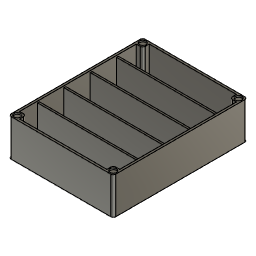
Wingspan - Food Tokens Container (Autodesk Fusion 360 design; units mm, degrees)
Autodesk Fusion 360 part; units mm, degrees
sketch "Skizze1" plane through (0, 0, 0) normal (0, 0, 1) x (1, 0, 0)
  line L0 (0, 0) -> (85, 0)
  line L1 (85, 0) -> (85, 109)
  line L2 (85, 109) -> (0, 109)
  line L3 (0, 109) -> (0, 0)
  dimension "d1" = 85
  dimension "d2" = 109
  constraint horizontal L0
  constraint vertical L1
  constraint horizontal L2
  constraint vertical L3
  constraint coincident L0.start L3.end
  measures "d1" distance of L0.start L0.end
  measures "d2" distance of L0.start L2.end
extrude "Extrusion11" add sketch "Skizze1" along normal blind 30
sketch "Skizze7" plane through (0, 0, 30) normal (0, 0, 1) x (-1, 0, 0)
  line L0 (0, -109) -> (0, 0)
  line L1 (0, 0) -> (-85, 0)
  line L2 (-85, 0) -> (-85, -109)
  line L3 (-85, -109) -> (0, -109)
  line L4 (0, -109) -> (-7, -109)
  line L5 (-7, -109) -> (-7, -102)
  line L6 (-7, -102) -> (0, -102)
  line L7 (0, -102) -> (0, -109)
  line L8 (-85, -109) -> (-78, -109)
  line L9 (-78, -109) -> (-78, -102)
  line L10 (-78, -102) -> (-85, -102)
  line L11 (-85, -102) -> (-85, -109)
  line L12 (0, 0) -> (-7, 0)
  line L13 (-7, 0) -> (-7, -7)
  line L14 (-7, -7) -> (0, -7)
  line L15 (0, -7) -> (0, 0)
  line L16 (-85, 0) -> (-78, 0)
  line L17 (-78, 0) -> (-78, -7)
  line L18 (-78, -7) -> (-85, -7)
  line L19 (-85, -7) -> (-85, 0)
  circle A0 centre (-3.5, -3.5) radius 2.65
  circle A1 centre (-81.5, -3.5) radius 2.65
  circle A2 centre (-81.5, -105.5) radius 2.65
  circle A3 centre (-3.5, -105.5) radius 2.65
  dimension "d103" = 7
  dimension "d104" = 7
  dimension "d105" = 7
  dimension "d106" = 7
  dimension "d107" = 7
  dimension "d108" = 7
  dimension "d109" = 7
  dimension "d110" = 7
  dimension "d111" = 5.3
  dimension "d112" = 5.3
  dimension "d113" = 5.3
  dimension "d114" = 5.3
  dimension "d115" = 3.5
  dimension "d116" = 3.5
  dimension "d117" = 3.5
  dimension "d118" = 3.5
  dimension "d119" = 3.5
  dimension "d120" = 3.5
  dimension "d121" = 3.5
  dimension "d122" = 3.5
  constraint horizontal L4
  constraint vertical L5
  constraint horizontal L6
  constraint vertical L7
  constraint coincident L0.start L3.end
  constraint horizontal L8
  constraint vertical L9
  constraint horizontal L10
  constraint vertical L11
  constraint coincident L2.end L3.start
  constraint horizontal L12
  constraint vertical L13
  constraint horizontal L14
  constraint vertical L15
  constraint coincident L0.end L1.start
  constraint horizontal L16
  constraint vertical L17
  constraint horizontal L18
  constraint vertical L19
  constraint coincident L1.end L2.start
  measures "d103" distance of L0.start L4.end
  measures "d104" distance of L0.start L6.end
  measures "d105" distance of L2.end L8.end
  measures "d106" distance of L2.end L10.end
  measures "d107" distance of L0.end L12.end
  measures "d108" distance of L0.end L14.end
  measures "d109" distance of L1.end L16.end
  measures "d110" distance of L1.end L18.end
  measures "d111" diameter of A0
  measures "d112" diameter of A1
  measures "d113" diameter of A2
  measures "d114" diameter of A3
  measures "d115" distance of L7 A3.centre
  measures "d116" distance of L4 A3.centre
  measures "d117" distance of L11 A2.centre
  measures "d118" distance of L8 A2.centre
  measures "d119" distance of L19 A1.centre
  measures "d120" distance of L18 A1.centre
  measures "d121" distance of L14 A0.centre
  measures "d122" distance of L15 A0.centre
extrude "Extrusion12" cut sketch "Skizze7" against normal blind 1.2 contours A0 | A1 | A2 | A3
sketch "Skizze8" plane through (0, 0, 30) normal (0, 0, 1) x (-1, 0, 0)
  circle A0 centre (-81.5, -3.5) radius 2.65
  circle A1 centre (-3.5, -105.5) radius 2.65
  circle A2 centre (-3.5, -3.5) radius 2.65
  circle A3 centre (-81.5, -105.5) radius 2.65
  line L0 (0, -109) -> (0, 0)
  line L1 (0, 0) -> (-85, 0)
  line L2 (-85, 0) -> (-85, -109)
  line L3 (-85, -109) -> (0, -109)
  line L4 (-7, -1.75) -> (-78, -1.75)
  line L5 (-78, -1.75) -> (-78, -107.25)
  line L6 (-78, -107.25) -> (-7, -107.25)
  line L7 (-7, -107.25) -> (-7, -1.75)
  line L8 (-85, -109) -> (0, -109)
  line L9 (-7, -102) -> (-1.75, -102)
  line L10 (-1.75, -102) -> (-1.75, -7)
  line L11 (-1.75, -7) -> (-7, -7)
  line L12 (-7, -7) -> (-7, -102)
  line L13 (0, 0) -> (-7, 0)
  line L14 (0, -109) -> (-7, -109)
  line L15 (-78, -7) -> (-83.25, -7)
  line L16 (-83.25, -7) -> (-83.25, -102)
  line L17 (-83.25, -102) -> (-78, -102)
  line L18 (-78, -102) -> (-78, -7)
  line L19 (-85, 0) -> (-85, -109)
  line L20 (-85, -109) -> (-78, -109)
  line L21 (-85, 0) -> (-78, 0)
  dimension "d125" = 1.75
  dimension "d126" = 7
  dimension "d127" = 7
  dimension "d128" = 1.75
  dimension "d129" = 1.75
  dimension "d130" = 7
  dimension "d131" = 7
  dimension "d132" = 1.75
  dimension "d133" = 7
  dimension "d134" = 7
  constraint horizontal L4
  constraint vertical L5
  constraint horizontal L6
  constraint vertical L7
  constraint horizontal L9
  constraint vertical L10
  constraint horizontal L11
  constraint vertical L12
  constraint coincident L7 L9.start
  constraint horizontal L15
  constraint vertical L16
  constraint horizontal L17
  constraint vertical L18
  constraint coincident L5 L15.start
  measures "d125" distance of L1 L4
  measures "d126" distance of L0 L7
  measures "d127" distance of L2 L5
  measures "d128" distance of L6 L8
  measures "d129" distance of L0 L10
  measures "d130" distance of L11 L13
  measures "d131" distance of L9 L14
  measures "d132" distance of L16 L19
  measures "d133" distance of L17 L20
  measures "d134" distance of L15 L21
extrude "Extrusion13" cut sketch "Skizze8" against normal blind 28.25 contours L4 L5 L6 L7 L12 L18 | L7 L9 L10 L11 L12 | L5 L15 L16 L17 L18
sketch "Skizze9" plane through (0, 0, 0) normal (0, 0, -1) x (1, 0, 0)
  line L0 (0, 0) -> (0, -109)
  line L1 (0, -109) -> (85, -109)
  line L2 (85, -109) -> (85, 0)
  line L3 (85, 0) -> (0, 0)
  line L4 (0, 0) -> (7, 0)
  line L5 (7, 0) -> (7, -7)
  line L6 (7, -7) -> (0, -7)
  line L7 (0, -7) -> (0, 0)
  line L8 (85, 0) -> (78, 0)
  line L9 (78, 0) -> (78, -7)
  line L10 (78, -7) -> (85, -7)
  line L11 (85, -7) -> (85, 0)
  line L12 (85, -109) -> (78, -109)
  line L13 (78, -109) -> (78, -102)
  line L14 (78, -102) -> (85, -102)
  line L15 (85, -102) -> (85, -109)
  line L16 (0, -109) -> (7, -109)
  line L17 (7, -109) -> (7, -102)
  line L18 (7, -102) -> (0, -102)
  line L19 (0, -102) -> (0, -109)
  circle A0 centre (3.5, -105.5) radius 2.65
  circle A1 centre (81.5, -105.5) radius 2.65
  circle A2 centre (81.5, -3.5) radius 2.65
  circle A3 centre (3.5, -3.5) radius 2.65
  dimension "d137" = 7
  dimension "d138" = 7
  dimension "d139" = 7
  dimension "d140" = 7
  dimension "d141" = 7
  dimension "d142" = 7
  dimension "d143" = 7
  dimension "d144" = 7
  dimension "d145" = 5.3
  dimension "d146" = 3.5
  dimension "d147" = 3.5
  dimension "d148" = 5.3
  dimension "d149" = 3.5
  dimension "d150" = 3.5
  dimension "d151" = 5.3
  dimension "d152" = 3.5
  dimension "d153" = 3.5
  dimension "d154" = 5.3
  dimension "d155" = 3.5
  dimension "d156" = 3.5
  constraint horizontal L4
  constraint vertical L5
  constraint horizontal L6
  constraint vertical L7
  constraint coincident L0.start L3.end
  constraint horizontal L8
  constraint vertical L9
  constraint horizontal L10
  constraint vertical L11
  constraint coincident L2.end L3.start
  constraint horizontal L12
  constraint vertical L13
  constraint horizontal L14
  constraint vertical L15
  constraint coincident L1.end L2.start
  constraint horizontal L16
  constraint vertical L17
  constraint horizontal L18
  constraint vertical L19
  constraint coincident L0.end L1.start
  measures "d137" distance of L0.start L4.end
  measures "d138" distance of L0.start L6.end
  measures "d139" distance of L2.end L8.end
  measures "d140" distance of L2.end L10.end
  measures "d141" distance of L1.end L12.end
  measures "d142" distance of L1.end L14.end
  measures "d143" distance of L0.end L16.end
  measures "d144" distance of L0.end L18.end
  measures "d145" diameter of A0
  measures "d146" distance of L16 A0.centre
  measures "d147" distance of L19 A0.centre
  measures "d148" diameter of A1
  measures "d149" distance of L12 A1.centre
  measures "d150" distance of L15 A1.centre
  measures "d151" diameter of A2
  measures "d152" distance of L11 A2.centre
  measures "d153" distance of L8 A2.centre
  measures "d154" diameter of A3
  measures "d155" distance of L4 A3.centre
  measures "d156" distance of L7 A3.centre
extrude "Extrusion14" cut sketch "Skizze9" against normal blind 1.2 contours A0 | A1 | A2 | A3
sketch "Skizze10" plane through (0, 0, 1.75) normal (0, 0, 1) x (-1, 0, 0)
  line L0 (-83.25, -102) -> (-78, -102)
  line L1 (-78, -102) -> (-78, -107.25)
  line L2 (-78, -107.25) -> (-7, -107.25)
  line L3 (-7, -107.25) -> (-7, -102)
  line L4 (-7, -102) -> (-1.75, -102)
  line L5 (-1.75, -102) -> (-1.75, -7)
  line L6 (-1.75, -7) -> (-7, -7)
  line L7 (-7, -7) -> (-7, -1.75)
  line L8 (-7, -1.75) -> (-78, -1.75)
  line L9 (-78, -1.75) -> (-78, -7)
  line L10 (-78, -7) -> (-83.25, -7)
  line L11 (-83.25, -7) -> (-83.25, -102)
  line L12 (-83.25, -87.35) -> (-1.75, -87.35)
  line L13 (-1.75, -87.35) -> (-1.75, -85.85)
  line L14 (-1.75, -85.85) -> (-83.25, -85.85)
  line L15 (-83.25, -85.85) -> (-83.25, -87.35)
  line L16 (-83.25, -65.95) -> (-1.75, -65.95)
  line L17 (-1.75, -65.95) -> (-1.75, -64.45)
  line L18 (-1.75, -64.45) -> (-83.25, -64.45)
  line L19 (-83.25, -64.45) -> (-83.25, -65.95)
  line L20 (-83.25, -44.55) -> (-1.75, -44.55)
  line L21 (-1.75, -44.55) -> (-1.75, -43.05)
  line L22 (-1.75, -43.05) -> (-83.25, -43.05)
  line L23 (-83.25, -43.05) -> (-83.25, -44.55)
  line L24 (-83.25, -23.15) -> (-1.75, -23.15)
  line L25 (-1.75, -23.15) -> (-1.75, -21.65)
  line L26 (-1.75, -21.65) -> (-83.25, -21.65)
  line L27 (-83.25, -21.65) -> (-83.25, -23.15)
  dimension "d159" = 1.5
  dimension "d160" = 19.9
  dimension "d161" = 1.5
  dimension "d162" = 19.9
  dimension "d163" = 1.5
  dimension "d164" = 19.9
  dimension "d165" = 1.5
  dimension "d166" = 19.9
  constraint horizontal L12
  constraint vertical L13
  constraint horizontal L14
  constraint vertical L15
  constraint coincident L5 L13.end
  constraint coincident L11 L12.start
  constraint horizontal L16
  constraint vertical L17
  constraint horizontal L18
  constraint vertical L19
  constraint coincident L5 L17.end
  constraint coincident L11 L16.start
  constraint horizontal L20
  constraint vertical L21
  constraint horizontal L22
  constraint vertical L23
  constraint coincident L5 L21.end
  constraint coincident L11 L20.start
  constraint horizontal L24
  constraint vertical L25
  constraint horizontal L26
  constraint vertical L27
  constraint coincident L5 L25.end
  constraint coincident L11 L24.start
  measures "d159" distance of L12 L14
  measures "d160" distance of L2 L12
  measures "d161" distance of L16 L18
  measures "d162" distance of L14 L16
  measures "d163" distance of L20 L22
  measures "d164" distance of L18 L20
  measures "d165" distance of L24 L26
  measures "d166" distance of L22 L24
extrude "Extrusion15" add sketch "Skizze10" along normal blind 27 contours L5 L11 L12 L13 L14 L15 | L5 L11 L16 L17 L18 L19 | L5 L11 L20 L21 L22 L23 | L5 L11 L24 L25 L26 L27
fillet "Abrundung4" radius 2 8 edges at (0, 109, 15) (0, 0, 15) (85, 0, 15) (85, 109, 15) (7, 102, 15.875) (7, 7, 15.875) (78, 7, 15.875) (78, 102, 15.875)
sketch "Skizze11" plane through (0, 0, 1.75) normal (0, 0, 1) x (-1, 0, 0)
  line L0 (-83.25, -21.65) -> (-1.75, -21.65)
  line L1 (-1.75, -21.65) -> (-1.75, -7)
  line L2 (-1.75, -7) -> (-5, -7)
  arc A0 (-7, -5) -> (-5, -7) centre (-5, -5) ccw
  line L3 (-7, -5) -> (-7, -1.75)
  line L4 (-7, -1.75) -> (-78, -1.75)
  line L5 (-78, -1.75) -> (-78, -5)
  arc A1 (-80, -7) -> (-78, -5) centre (-80, -5) ccw
  line L6 (-80, -7) -> (-83.25, -7)
  line L7 (-83.25, -7) -> (-83.25, -21.65)
  spline S0 degree 3 poles (-39.178, -19.5242) (-39.2616, -19.4406) (-39.167, -18.9822) (-38.9679, -18.5054) knots 0 0 0 0 1 1 1 1
  line L8 (-38.9679, -18.5054) -> (-38.6057, -17.6386)
  line L9 (-38.6057, -17.6386) -> (-39.8375, -16.3539)
  spline S1 degree 3 poles (-39.8375, -16.3539) (-41.1646, -14.9699) (-42.027, -14.6539) (-44.5452, -14.6292) knots 0 0 0 0 1 1 1 1
  spline S2 degree 3 poles (-44.5452, -14.6292) (-48.426, -14.5911) (-50.326, -12.4607) (-50.3212, -8.1525) knots 0 0 0 0 1 1 1 1
  spline S3 degree 3 poles (-50.3212, -8.1525) (-50.3184, -5.5992) (-49.8967, -4.7798) (-48.5851, -4.7798) knots 0 0 0 0 1 1 1 1
  spline S4 degree 3 poles (-48.5851, -4.7798) (-47.4873, -4.7798) (-47.295, -5.142) (-47.1328, -7.5151) knots 0 0 0 0 1 1 1 1
  spline S5 degree 3 poles (-47.1328, -7.5151) (-47.0433, -8.8234) (-46.8587, -9.5644) (-46.5038, -10.0381) knots 0 0 0 0 1 1 1 1
  spline S6 degree 3 poles (-46.5038, -10.0381) (-46.014, -10.6921) (-45.9327, -10.709) (-43.2549, -10.7115) knots 0 0 0 0 1 1 1 1
  spline S7 degree 3 poles (-43.2549, -10.7115) (-40.9745, -10.7136) (-40.3063, -10.8069) (-39.3182, -11.2613) knots 0 0 0 0 1 1 1 1
  spline S8 degree 3 poles (-39.3182, -11.2613) (-38.0099, -11.8629) (-35.6932, -13.8922) (-35.4539, -14.6461) knots 0 0 0 0 1 1 1 1
  spline S9 degree 3 poles (-35.4539, -14.6461) (-35.335, -15.0207) (-35.0599, -15.1242) (-34.1837, -15.1242) knots 0 0 0 0 1 1 1 1
  spline S10 degree 3 poles (-34.1837, -15.1242) (-33.3782, -15.1242) (-33.0654, -15.2259) (-33.0654, -15.4878) knots 0 0 0 0 1 1 1 1
  spline S11 degree 3 poles (-33.0654, -15.4878) (-33.0654, -15.9956) (-33.5581, -16.2462) (-33.8947, -15.9096) knots 0 0 0 0 1 1 1 1
  spline S12 degree 3 poles (-33.8947, -15.9096) (-34.2764, -15.5279) (-35.3348, -15.5533) (-35.3417, -15.9442) knots 0 0 0 0 1 1 1 1
  spline S13 degree 3 poles (-35.3417, -15.9442) (-35.3541, -16.6404) (-36.2962, -17.4664) (-37.255, -17.6217) knots 0 0 0 0 1 1 1 1
  spline S14 degree 3 poles (-37.255, -17.6217) (-38.1386, -17.7648) (-38.2503, -17.8673) (-38.3638, -18.6401) knots 0 0 0 0 1 1 1 1
  spline S15 degree 3 poles (-38.3638, -18.6401) (-38.4838, -19.4576) (-38.8486, -19.8537) (-39.178, -19.5242) knots 0 0 0 0 1 1 1 1
  spline S16 degree 3 poles (-48.0381, -37.5695) (-47.8963, -37.326) (-47.5089, -37.1504) (-47.1139, -37.1504) knots 0 0 0 0 1 1 1 1
  spline S17 degree 3 poles (-47.1139, -37.1504) (-46.1113, -37.1504) (-45.5008, -37.8028) (-44.8901, -39.527) knots 0 0 0 0 1 1 1 1
  spline S18 degree 3 poles (-44.8901, -39.527) (-44.5903, -40.3731) (-44.2177, -41.1071) (-44.062, -41.1581) knots 0 0 0 0 1 1 1 1
  spline S19 degree 3 poles (-44.062, -41.1581) (-43.5866, -41.3138) (-43.2627, -40.3632) (-43.4171, -39.2653) knots 0 0 0 0 1 1 1 1
  spline S20 degree 3 poles (-43.4171, -39.2653) (-43.5316, -38.4508) (-43.7224, -38.1252) (-44.3057, -37.7491) knots 0 0 0 0 1 1 1 1
  spline S21 degree 3 poles (-44.3057, -37.7491) (-45.5367, -36.9552) (-46.1328, -35.6221) (-46.1374, -33.653) knots 0 0 0 0 1 1 1 1
  spline S22 degree 3 poles (-46.1374, -33.653) (-46.1395, -32.7173) (-46.0712, -31.281) (-45.9855, -30.4612) knots 0 0 0 0 1 1 1 1
  spline S23 degree 3 poles (-45.9855, -30.4612) (-45.8497, -29.1622) (-45.7724, -28.9856) (-45.3837, -29.0873) knots 0 0 0 0 1 1 1 1
  spline S24 degree 3 poles (-45.3837, -29.0873) (-44.801, -29.2397) (-44.6054, -28.8388) (-44.089, -26.4331) knots 0 0 0 0 1 1 1 1
  spline S25 degree 3 poles (-44.089, -26.4331) (-43.7861, -25.0222) (-43.5619, -24.4573) (-43.3046, -24.4573) knots 0 0 0 0 1 1 1 1
  spline S26 degree 3 poles (-43.3046, -24.4573) (-43.1065, -24.4573) (-42.128, -25.2386) (-41.1301, -26.1936) knots 0 0 0 0 1 1 1 1
  spline S27 degree 3 poles (-41.1301, -26.1936) (-39.2398, -28.0026) (-38.815, -28.9068) (-39.874, -28.8668) knots 0 0 0 0 1 1 1 1
  spline S28 degree 3 poles (-39.874, -28.8668) (-40.3813, -28.8476) (-40.4184, -28.9198) (-40.2801, -29.6571) knots 0 0 0 0 1 1 1 1
  spline S29 degree 3 poles (-40.2801, -29.6571) (-40.1963, -30.1034) (-39.8643, -30.9641) (-39.5422, -31.5699) knots 0 0 0 0 1 1 1 1
  spline S30 degree 3 poles (-39.5422, -31.5699) (-38.8325, -32.9048) (-38.7828, -34.4696) (-39.4067, -35.8431) knots 0 0 0 0 1 1 1 1
  spline S31 degree 3 poles (-39.4067, -35.8431) (-39.916, -36.9641) (-41.1366, -38.0773) (-42.0588, -38.2618) knots 0 0 0 0 1 1 1 1
  spline S32 degree 3 poles (-42.0588, -38.2618) (-42.6091, -38.3718) (-42.6849, -38.4878) (-42.5972, -39.0857) knots 0 0 0 0 1 1 1 1
  spline S33 degree 3 poles (-42.5972, -39.0857) (-42.4138, -40.3352) (-42.7591, -41.4619) (-43.4, -41.7056) knots 0 0 0 0 1 1 1 1
  spline S34 degree 3 poles (-43.4, -41.7056) (-44.4841, -42.1177) (-45.0821, -41.6481) (-45.6512, -39.9379) knots 0 0 0 0 1 1 1 1
  spline S35 degree 3 poles (-45.6512, -39.9379) (-46.2604, -38.1073) (-46.6824, -37.6428) (-47.355, -38.0629) knots 0 0 0 0 1 1 1 1
  spline S36 degree 3 poles (-47.355, -38.0629) (-48.2118, -38.598) (-48.5112, -38.3817) (-48.0381, -37.5695) knots 0 0 0 0 1 1 1 1
sketch "Skizze12" plane through (0, 0, 1.75) normal (0, 0, 1) x (-1, 0, 0)
  line L0 (-1.75, -44.55) -> (-83.25, -44.55)
  line L1 (-83.25, -44.55) -> (-83.25, -64.45)
  line L2 (-83.25, -64.45) -> (-1.75, -64.45)
  line L3 (-1.75, -64.45) -> (-1.75, -44.55)
  spline S0 degree 3 poles (-49.7706, -52.9271) (-49.2736, -51.3545) (-48.2065, -50.5145) (-46.7263, -50.5306) knots 0 0 0 0 1 1 1 1
  spline S1 degree 3 poles (-46.7263, -50.5306) (-45.7005, -50.5418) (-44.2379, -51.4293) (-43.9023, -52.2442) knots 0 0 0 0 1 1 1 1
  spline S2 degree 3 poles (-43.9023, -52.2442) (-43.6832, -52.7759) (-43.4579, -52.8987) (-42.4991, -53.0086) knots 0 0 0 0 1 1 1 1
  spline S3 degree 3 poles (-42.4991, -53.0086) (-41.8709, -53.0806) (-41.1277, -53.2147) (-40.8474, -53.3066) knots 0 0 0 0 1 1 1 1
  spline S4 degree 3 poles (-40.8474, -53.3066) (-40.4432, -53.4391) (-40.3494, -53.4082) (-40.3937, -53.157) knots 0 0 0 0 1 1 1 1
  spline S5 degree 3 poles (-40.3937, -53.157) (-40.4245, -52.9828) (-40.7763, -52.7679) (-41.1755, -52.6793) knots 0 0 0 0 1 1 1 1
  spline S6 degree 3 poles (-41.1755, -52.6793) (-42.9496, -52.286) (-43.954, -50.4074) (-43.2546, -48.7907) knots 0 0 0 0 1 1 1 1
  spline S7 degree 3 poles (-43.2546, -48.7907) (-42.4335, -46.8925) (-40.0051, -46.522) (-38.6625, -48.0901) knots 0 0 0 0 1 1 1 1
  spline S8 degree 3 poles (-38.6625, -48.0901) (-37.654, -49.268) (-37.9063, -51.2765) (-39.1693, -52.1244) knots 0 0 0 0 1 1 1 1
  spline S9 degree 3 poles (-39.1693, -52.1244) (-40.1579, -52.7881) (-39.8896, -53.4953) (-38.2085, -54.6568) knots 0 0 0 0 1 1 1 1
  spline S10 degree 3 poles (-38.2085, -54.6568) (-36.6829, -55.7109) (-34.4155, -58.5444) (-34.5488, -59.2304) knots 0 0 0 0 1 1 1 1
  spline S11 degree 3 poles (-34.5488, -59.2304) (-34.7584, -60.3092) (-35.9602, -59.9491) (-36.1778, -58.7423) knots 0 0 0 0 1 1 1 1
  spline S12 degree 3 poles (-36.1778, -58.7423) (-36.2345, -58.4273) (-36.6207, -57.6838) (-37.0358, -57.0901) knots 0 0 0 0 1 1 1 1
  spline S13 degree 3 poles (-37.0358, -57.0901) (-37.6472, -56.216) (-37.8956, -56.0292) (-38.3427, -56.108) knots 0 0 0 0 1 1 1 1
  spline S14 degree 3 poles (-38.3427, -56.108) (-39.3574, -56.287) (-39.5439, -56.5254) (-39.2742, -57.2992) knots 0 0 0 0 1 1 1 1
  spline S15 degree 3 poles (-39.2742, -57.2992) (-38.7276, -58.8673) (-39.8079, -60.5236) (-41.5812, -60.8363) knots 0 0 0 0 1 1 1 1
  spline S16 degree 3 poles (-41.5812, -60.8363) (-42.3513, -60.9721) (-42.6827, -60.8888) (-43.4169, -60.3747) knots 0 0 0 0 1 1 1 1
  spline S17 degree 3 poles (-43.4169, -60.3747) (-44.206, -59.8222) (-44.3372, -59.6086) (-44.5181, -58.5827) knots 0 0 0 0 1 1 1 1
  spline S18 degree 3 poles (-44.5181, -58.5827) (-44.699, -57.5567) (-44.6487, -57.3112) (-44.0962, -56.522) knots 0 0 0 0 1 1 1 1
  spline S19 degree 3 poles (-44.0962, -56.522) (-43.561, -55.7578) (-43.3145, -55.599) (-42.4179, -55.4409) knots 0 0 0 0 1 1 1 1
  spline S20 degree 3 poles (-42.4179, -55.4409) (-41.7308, -55.3197) (-41.1571, -55.3679) (-40.7612, -55.5801) knots 0 0 0 0 1 1 1 1
  spline S21 degree 3 poles (-40.7612, -55.5801) (-40.1874, -55.8876) (-39.1508, -55.7318) (-38.9839, -55.3129) knots 0 0 0 0 1 1 1 1
  spline S22 degree 3 poles (-38.9839, -55.3129) (-38.8763, -55.0427) (-40.8372, -54.2918) (-42.1581, -54.0974) knots 0 0 0 0 1 1 1 1
  spline S23 degree 3 poles (-42.1581, -54.0974) (-43.079, -53.9618) (-43.3643, -53.9892) (-43.398, -54.2163) knots 0 0 0 0 1 1 1 1
  spline S24 degree 3 poles (-43.398, -54.2163) (-43.4976, -54.8884) (-44.5427, -56.2674) (-45.2338, -56.639) knots 0 0 0 0 1 1 1 1
  spline S25 degree 3 poles (-45.2338, -56.639) (-47.6852, -57.957) (-50.6052, -55.5679) (-49.7706, -52.9271) knots 0 0 0 0 1 1 1 1
  spline S26 degree 3 poles (-45.2787, -74.9924) (-44.9999, -74.3782) (-44.3971, -73.3538) (-43.9391, -72.716) knots 0 0 0 0 1 1 1 1
  line L4 (-43.9391, -72.716) -> (-43.1064, -71.5565)
  line L5 (-43.1064, -71.5565) -> (-43.5424, -70.1731)
  spline S27 degree 3 poles (-43.5424, -70.1731) (-44.2718, -67.8593) (-44.0313, -66.6033) (-43.0637, -67.6725) knots 0 0 0 0 1 1 1 1
  spline S28 degree 3 poles (-43.0637, -67.6725) (-42.5023, -68.2929) (-42.1203, -68.313) (-41.0839, -67.7771) knots 0 0 0 0 1 1 1 1
  spline S29 degree 3 poles (-41.0839, -67.7771) (-40.6491, -67.5523) (-40.2288, -67.4329) (-40.1499, -67.5118) knots 0 0 0 0 1 1 1 1
  spline S30 degree 3 poles (-40.1499, -67.5118) (-40.071, -67.5907) (-40.1556, -68.5272) (-40.3379, -69.593) knots 0 0 0 0 1 1 1 1
  line L6 (-40.3379, -69.593) -> (-40.6694, -71.5307)
  line L7 (-40.6694, -71.5307) -> (-39.7598, -72.7808)
  spline S31 degree 3 poles (-39.7598, -72.7808) (-38.2243, -74.8911) (-37.9219, -75.6887) (-37.9067, -77.6678) knots 0 0 0 0 1 1 1 1
  spline S32 degree 3 poles (-37.9067, -77.6678) (-37.8949, -79.2054) (-38.0106, -79.7016) (-38.6555, -80.8806) knots 0 0 0 0 1 1 1 1
  spline S33 degree 3 poles (-38.6555, -80.8806) (-39.365, -82.1775) (-41.7036, -84.5519) (-42.2715, -84.5519) knots 0 0 0 0 1 1 1 1
  spline S34 degree 3 poles (-42.2715, -84.5519) (-42.9562, -84.5519) (-44.5428, -83.07) (-45.1389, -81.8738) knots 0 0 0 0 1 1 1 1
  spline S35 degree 3 poles (-45.1389, -81.8738) (-46.0018, -80.1421) (-46.071, -76.7381) (-45.2787, -74.9924) knots 0 0 0 0 1 1 1 1
  spline S36 degree 3 poles (-42.1284, -81.8819) (-41.7713, -82.2389) (-41.121, -82.026) (-41.121, -81.552) knots 0 0 0 0 1 1 1 1
  spline S37 degree 3 poles (-41.121, -81.552) (-41.121, -81.0956) (-41.571, -80.8328) (-42.0426, -81.0137) knots 0 0 0 0 1 1 1 1
  spline S38 degree 3 poles (-42.0426, -81.0137) (-42.4946, -81.1872) (-42.5241, -81.4862) (-42.1284, -81.8819) knots 0 0 0 0 1 1 1 1
sketch "Skizze13" plane through (0, 0, 1.75) normal (0, 0, 1) x (-1, 0, 0)
  line L0 (-1.75, -87.35) -> (-83.25, -87.35)
  line L1 (-83.25, -87.35) -> (-83.25, -102)
  line L2 (-83.25, -102) -> (-80, -102)
  arc A0 (-78, -104) -> (-80, -102) centre (-80, -104) ccw
  line L3 (-78, -104) -> (-78, -107.25)
  line L4 (-78, -107.25) -> (-7, -107.25)
  line L5 (-7, -107.25) -> (-7, -104)
  arc A1 (-5, -102) -> (-7, -104) centre (-5, -104) ccw
  line L6 (-5, -102) -> (-1.75, -102)
  line L7 (-1.75, -102) -> (-1.75, -87.35)
  spline S0 degree 3 poles (-33.401, -102.4774) (-34.0318, -102.0189) (-34.2592, -101.9971) (-35.0353, -102.3208) knots 0 0 0 0 1 1 1 1
  spline S1 degree 3 poles (-35.0353, -102.3208) (-36.1056, -102.7672) (-38.3354, -102.528) (-39.4305, -101.8493) knots 0 0 0 0 1 1 1 1
  line L8 (-39.4305, -101.8493) -> (-40.1458, -101.406)
  line L9 (-40.1458, -101.406) -> (-38.1867, -100.881)
  spline S2 degree 3 poles (-38.1867, -100.881) (-36.2327, -100.3575) (-36.2228, -100.358) (-34.475, -101.092) knots 0 0 0 0 1 1 1 1
  spline S3 degree 3 poles (-34.475, -101.092) (-32.4787, -101.9304) (-32.0923, -102.2319) (-32.4299, -102.6879) knots 0 0 0 0 1 1 1 1
  spline S4 degree 3 poles (-32.4299, -102.6879) (-32.5992, -102.9166) (-32.8808, -102.8556) (-33.401, -102.4774) knots 0 0 0 0 1 1 1 1
  spline S5 degree 3 poles (-34.6284, -100.4502) (-36.058, -99.4522) (-36.6114, -98.6882) (-37.3901, -96.6379) knots 0 0 0 0 1 1 1 1
  spline S6 degree 3 poles (-37.3901, -96.6379) (-37.7956, -95.5701) (-38.1075, -94.6601) (-38.0831, -94.6156) knots 0 0 0 0 1 1 1 1
  spline S7 degree 3 poles (-38.0831, -94.6156) (-37.9666, -94.403) (-35.044, -97.0939) (-34.3569, -98.0465) knots 0 0 0 0 1 1 1 1
  spline S8 degree 3 poles (-34.3569, -98.0465) (-33.4338, -99.326) (-33.2711, -99.8255) (-33.5461, -100.5353) knots 0 0 0 0 1 1 1 1
  spline S9 degree 3 poles (-33.5461, -100.5353) (-33.7374, -101.029) (-33.8073, -101.0235) (-34.6284, -100.4502) knots 0 0 0 0 1 1 1 1
  spline S10 degree 3 poles (-42.0606, -100.4671) (-42.8045, -100.0162) (-43.4448, -99.5289) (-43.4835, -99.3843) knots 0 0 0 0 1 1 1 1
  spline S11 degree 3 poles (-43.4835, -99.3843) (-43.5307, -99.2083) (-42.6862, -98.9185) (-40.9283, -98.5074) knots 0 0 0 0 1 1 1 1
  spline S12 degree 3 poles (-40.9283, -98.5074) (-38.0758, -97.8403) (-37.9785, -97.8618) (-36.7534, -99.4276) knots 0 0 0 0 1 1 1 1
  line L10 (-36.7534, -99.4276) -> (-36.3163, -99.9861)
  line L11 (-36.3163, -99.9861) -> (-38.5123, -100.6365)
  line L12 (-38.5123, -100.6365) -> (-40.7082, -101.2869)
  line L13 (-40.7082, -101.2869) -> (-42.0606, -100.4671)
  spline S13 degree 3 poles (-44.1344, -98.5417) (-44.4508, -98.5029) (-45.1362, -98.0326) (-45.6575, -97.4965) knots 0 0 0 0 1 1 1 1
  line L14 (-45.6575, -97.4965) -> (-46.6054, -96.5219)
  line L15 (-46.6054, -96.5219) -> (-44.7858, -96.2242)
  spline S14 degree 3 poles (-44.7858, -96.2242) (-43.7851, -96.0605) (-42.663, -95.9561) (-42.2924, -95.9922) knots 0 0 0 0 1 1 1 1
  spline S15 degree 3 poles (-42.2924, -95.9922) (-41.5799, -96.0616) (-39.6518, -97.0303) (-39.5625, -97.3637) knots 0 0 0 0 1 1 1 1
  spline S16 degree 3 poles (-39.5625, -97.3637) (-39.4924, -97.6251) (-43.3996, -98.6319) (-44.1344, -98.5417) knots 0 0 0 0 1 1 1 1
  spline S17 degree 3 poles (-39.3341, -96.5948) (-40.7887, -95.7152) (-41.1922, -95.2003) (-41.5898, -93.7163) knots 0 0 0 0 1 1 1 1
  line L16 (-41.5898, -93.7163) -> (-41.8941, -92.5805)
  line L17 (-41.8941, -92.5805) -> (-40.6491, -93.2797)
  spline S18 degree 3 poles (-40.6491, -93.2797) (-39.286, -94.0452) (-38.5067, -95.0851) (-38.2787, -96.4432) knots 0 0 0 0 1 1 1 1
  line L18 (-38.2787, -96.4432) -> (-38.131, -97.3224)
  line L19 (-38.131, -97.3224) -> (-39.3341, -96.5948)
  spline S19 degree 3 poles (-42.6987, -95.1995) (-43.8807, -94.7687) (-44.7862, -93.6054) (-44.8571, -92.4266) knots 0 0 0 0 1 1 1 1
  line L20 (-44.8571, -92.4266) -> (-44.91, -91.5463)
  line L21 (-44.91, -91.5463) -> (-43.7921, -92.1555)
  spline S20 degree 3 poles (-43.7921, -92.1555) (-42.8087, -92.6914) (-42.6166, -92.931) (-42.1959, -94.146) knots 0 0 0 0 1 1 1 1
  spline S21 degree 3 poles (-42.1959, -94.146) (-41.9328, -94.9057) (-41.7282, -95.53) (-41.7412, -95.5335) knots 0 0 0 0 1 1 1 1
  spline S22 degree 3 poles (-41.7412, -95.5335) (-41.7542, -95.537) (-42.1851, -95.3867) (-42.6987, -95.1995) knots 0 0 0 0 1 1 1 1
  spline S23 degree 3 poles (-46.2014, -95.7592) (-46.7071, -95.7941) (-48.7205, -94.3722) (-48.547, -94.1026) knots 0 0 0 0 1 1 1 1
  spline S24 degree 3 poles (-48.547, -94.1026) (-48.5064, -94.0395) (-47.9081, -93.9826) (-47.2174, -93.9761) knots 0 0 0 0 1 1 1 1
  spline S25 degree 3 poles (-47.2174, -93.9761) (-46.0771, -93.9655) (-44.222, -94.6689) (-44.0899, -95.162) knots 0 0 0 0 1 1 1 1
  spline S26 degree 3 poles (-44.0899, -95.162) (-44.0358, -95.3637) (-45.1864, -95.6892) (-46.2014, -95.7592) knots 0 0 0 0 1 1 1 1
  spline S27 degree 3 poles (-46.0716, -93.3377) (-46.517, -93.1977) (-47.2561, -92.1625) (-47.4635, -91.3882) knots 0 0 0 0 1 1 1 1
  line L22 (-47.4635, -91.3882) -> (-47.6278, -90.7751)
  line L23 (-47.6278, -90.7751) -> (-46.7529, -91.1015)
  spline S28 degree 3 poles (-46.7529, -91.1015) (-46.0347, -91.3693) (-45.8317, -91.6003) (-45.6199, -92.3907) knots 0 0 0 0 1 1 1 1
  spline S29 degree 3 poles (-45.6199, -92.3907) (-45.3604, -93.3593) (-45.4442, -93.5349) (-46.0716, -93.3377) knots 0 0 0 0 1 1 1 1
  spline S30 degree 3 poles (-47.9846, -93.3622) (-48.3369, -93.3598) (-50.1216, -91.7416) (-49.8517, -91.6693) knots 0 0 0 0 1 1 1 1
  spline S31 degree 3 poles (-49.8517, -91.6693) (-49.7912, -91.6531) (-49.3167, -91.6971) (-48.7973, -91.7671) knots 0 0 0 0 1 1 1 1
  spline S32 degree 3 poles (-48.7973, -91.7671) (-48.0122, -91.8729) (-47.8191, -92.0205) (-47.6527, -92.6416) knots 0 0 0 0 1 1 1 1
  spline S33 degree 3 poles (-47.6527, -92.6416) (-47.5425, -93.0526) (-47.4834, -93.3835) (-47.5213, -93.3769) knots 0 0 0 0 1 1 1 1
  spline S34 degree 3 poles (-47.5213, -93.3769) (-47.5591, -93.3703) (-47.7676, -93.3637) (-47.9846, -93.3622) knots 0 0 0 0 1 1 1 1
extrude "Extrusion16" cut sketch "Skizze12" sketch "Skizze13" sketch "Skizze11" against normal blind 0.4 contours S0 S1 S2 S3 S4 S5 S6 S7 S8 S9 S10 S11 S12 S13 S14 S15 S16 S17 S18 S19 S20 S21 S22 S23 S24 S25 | S26 L4 L5 S27 S28 S29 S30 L6 L7 S31 S32 S33 S34 S35 of sketch 2 contours S0 S1 L8 L9 S2 S3 S4 | S5 S6 S7 S8 S9 | S10 S11 S12 L10 L11 L12 L13 | S13 L14 L15 S14 S15 S16 | S17 L16 L17 S18 L18 L19 | S19 L20 L21 S20 S21 S22 | S23 S24 S25 S26 | S27 L22 L23 S28 S29 | S30 S31 S32 S33 S34 of sketch 3 contours S0 L8 L9 S1 S2 S3 S4 S5 S6 S7 S8 S9 S10 S11 S12 S13 S14 S15 | S16 S17 S18 S19 S20 S21 S22 S23 S24 S25 S26 S27 S28 S29 S30 S31 S32 S33 S34 S35 S36
extrude "Extrusion5" [suppressed]
sketch "Skizze3" plane through (0, 0, 30) normal (0, 0, 1) x (-1, 0, 0)
  line L0 (0, -115) -> (0, 0)
  line L1 (0, 0) -> (-85, 0)
  line L2 (-85, 0) -> (-85, -115)
  line L3 (-85, -115) -> (0, -115)
  line L4 (0, -115) -> (-7, -115)
  line L5 (-7, -115) -> (-7, -108)
  line L6 (-7, -108) -> (0, -108)
  line L7 (0, -108) -> (0, -115)
  line L8 (-85, -115) -> (-78, -115)
  line L9 (-78, -115) -> (-78, -108)
  line L10 (-78, -108) -> (-85, -108)
  line L11 (-85, -108) -> (-85, -115)
  line L12 (-85, 0) -> (-78, 0)
  line L13 (-78, 0) -> (-78, -7)
  line L14 (-78, -7) -> (-85, -7)
  line L15 (-85, -7) -> (-85, 0)
  line L16 (0, 0) -> (-7, 0)
  line L17 (-7, 0) -> (-7, -7)
  line L18 (-7, -7) -> (0, -7)
  line L19 (0, -7) -> (0, 0)
  circle A0 centre (-3.5, -3.5) radius 2.65
  circle A1 centre (-81.5, -3.5) radius 2.65
  circle A2 centre (-81.5, -111.5) radius 2.65
  circle A3 centre (-3.5, -111.5) radius 2.65
  line L20 (-7, -113.25) -> (-78, -113.25)
  line L21 (-78, -113.25) -> (-78, -1.75)
  line L22 (-78, -1.75) -> (-7, -1.75)
  line L23 (-7, -1.75) -> (-7, -113.25)
  line L24 (-7, -108) -> (-1.75, -108)
  line L25 (-1.75, -108) -> (-1.75, -7)
  line L26 (-1.75, -7) -> (-7, -7)
  line L27 (-7, -7) -> (-7, -108)
  line L28 (-78, -108) -> (-83.25, -108)
  line L29 (-83.25, -108) -> (-83.25, -7)
  line L30 (-83.25, -7) -> (-78, -7)
  line L31 (-78, -7) -> (-78, -108)
  dimension "d45" = 7
  dimension "d46" = 7
  dimension "d47" = 7
  dimension "d48" = 7
  dimension "d49" = 7
  dimension "d50" = 7
  dimension "d51" = 7
  dimension "d52" = 7
  dimension "d53" = 5.3
  dimension "d54" = 3.5
  dimension "d55" = 3.5
  dimension "d56" = 5.3
  dimension "d57" = 3.5
  dimension "d58" = 3.5
  dimension "d59" = 5.3
  dimension "d60" = 3.5
  dimension "d61" = 3.5
  dimension "d62" = 5.3
  dimension "d63" = 3.5
  dimension "d64" = 3.5
  dimension "d65" = 1.75
  dimension "d66" = 1.75
  dimension "d67" = 1.75
  dimension "d68" = 1.75
  constraint horizontal L4
  constraint vertical L5
  constraint horizontal L6
  constraint vertical L7
  constraint coincident L0.start L3.end
  constraint horizontal L8
  constraint vertical L9
  constraint horizontal L10
  constraint vertical L11
  constraint coincident L2.end L3.start
  constraint horizontal L12
  constraint vertical L13
  constraint horizontal L14
  constraint vertical L15
  constraint coincident L1.end L2.start
  constraint horizontal L16
  constraint vertical L17
  constraint horizontal L18
  constraint vertical L19
  constraint coincident L0.end L1.start
  constraint horizontal L20
  constraint vertical L21
  constraint horizontal L22
  constraint vertical L23
  constraint coincident L13 L21.end
  constraint coincident L5 L20.start
  constraint horizontal L24
  constraint vertical L25
  constraint horizontal L26
  constraint vertical L27
  constraint coincident L18 L25.end
  constraint horizontal L28
  constraint vertical L29
  constraint horizontal L30
  constraint vertical L31
  constraint coincident L14 L29.end
  measures "d45" distance of L0.start L4.end
  measures "d46" distance of L0.start L6.end
  measures "d47" distance of L2.end L8.end
  measures "d48" distance of L2.end L10.end
  measures "d49" distance of L1.end L12.end
  measures "d50" distance of L1.end L14.end
  measures "d51" distance of L0.end L16.end
  measures "d52" distance of L0.end L18.end
  measures "d53" diameter of A0
  measures "d54" distance of L16 A0.centre
  measures "d55" distance of L17 A0.centre
  measures "d56" diameter of A1
  measures "d57" distance of L15 A1.centre
  measures "d58" distance of L14 A1.centre
  measures "d59" diameter of A2
  measures "d60" distance of L11 A2.centre
  measures "d61" distance of L10 A2.centre
  measures "d62" diameter of A3
  measures "d63" distance of L5 A3.centre
  measures "d64" distance of L6 A3.centre
  measures "d65" distance of L3 L20
  measures "d66" distance of L1 L22
  measures "d67" distance of L0 L25
  measures "d68" distance of L2 L29
extrude "Extrusion7" [suppressed]
extrude "Extrusion8" [suppressed]
sketch "Skizze5" plane through (0, 0, 0) normal (0, 0, -1) x (1, 0, 0)
  line L0 (0, 0) -> (0, -115)
  line L1 (0, -115) -> (85, -115)
  line L2 (85, -115) -> (85, 0)
  line L3 (85, 0) -> (0, 0)
  circle A0 centre (3.5, -111.5) radius 2.65
  circle A1 centre (81.5, -111.5) radius 2.65
  circle A2 centre (3.5, -3.5) radius 2.65
  circle A3 centre (81.5, -3.5) radius 2.65
  dimension "d73" = 5.3
  dimension "d74" = 3.5
  dimension "d75" = 3.5
  dimension "d76" = 5.3
  dimension "d77" = 3.5
  dimension "d78" = 3.5
  dimension "d79" = 5.3
  dimension "d80" = 3.5
  dimension "d81" = 3.5
  dimension "d82" = 5.3
  dimension "d83" = 3.5
  dimension "d84" = 3.5
  measures "d73" diameter of A0
  measures "d74" distance of L1 A0.centre
  measures "d75" distance of L0 A0.centre
  measures "d76" diameter of A1
  measures "d77" distance of L2 A1.centre
  measures "d78" distance of L1 A1.centre
  measures "d79" diameter of A2
  measures "d80" distance of L0 A2.centre
  measures "d81" distance of L3 A2.centre
  measures "d82" diameter of A3
  measures "d83" distance of L2 A3.centre
  measures "d84" distance of L3 A3.centre
extrude "Extrusion9" [suppressed]
sketch "Skizze6" plane through (0, 0, 1.75) normal (0, 0, 1) x (-1, 0, 0)
  line L0 (-7, -108) -> (-1.75, -108)
  line L1 (-1.75, -108) -> (-1.75, -7)
  line L2 (-1.75, -7) -> (-7, -7)
  line L3 (-7, -7) -> (-7, -1.75)
  line L4 (-7, -1.75) -> (-78, -1.75)
  line L5 (-78, -1.75) -> (-78, -7)
  line L6 (-78, -7) -> (-83.25, -7)
  line L7 (-83.25, -7) -> (-83.25, -108)
  line L8 (-83.25, -108) -> (-78, -108)
  line L9 (-78, -108) -> (-78, -113.25)
  line L10 (-78, -113.25) -> (-7, -113.25)
  line L11 (-7, -113.25) -> (-7, -108)
  line L12 (-83.25, -86.69) -> (-1.75, -86.69)
  line L13 (-1.75, -86.69) -> (-1.75, -84.94)
  line L14 (-1.75, -84.94) -> (-83.25, -84.94)
  line L15 (-83.25, -84.94) -> (-83.25, -86.69)
  line L16 (-83.25, -58.38) -> (-1.75, -58.38)
  line L17 (-1.75, -58.38) -> (-1.75, -56.63)
  line L18 (-1.75, -56.63) -> (-83.25, -56.63)
  line L19 (-83.25, -56.63) -> (-83.25, -58.38)
  line L20 (-83.25, -30.07) -> (-1.75, -30.07)
  line L21 (-1.75, -30.07) -> (-1.75, -28.32)
  line L22 (-1.75, -28.32) -> (-83.25, -28.32)
  line L23 (-83.25, -28.32) -> (-83.25, -30.07)
  dimension "d87" = 1.75
  dimension "d88" = 26.56
  dimension "d89" = 1.75
  dimension "d90" = 26.56
  dimension "d91" = 1.75
  dimension "d92" = 26.56
  constraint horizontal L12
  constraint vertical L13
  constraint horizontal L14
  constraint vertical L15
  constraint coincident L1 L13.end
  constraint coincident L7 L12.start
  constraint horizontal L16
  constraint vertical L17
  constraint horizontal L18
  constraint vertical L19
  constraint coincident L7 L16.start
  constraint horizontal L20
  constraint vertical L21
  constraint horizontal L22
  constraint vertical L23
  constraint coincident L7 L20.start
  measures "d87" distance of L12 L14
  measures "d88" distance of L10 L12
  measures "d89" distance of L16.start L18.end
  measures "d90" distance of L14 L16
  measures "d91" distance of L20.start L22.end
  measures "d92" distance of L18 L20
extrude "Extrusion10" [suppressed]
fillet "Abrundung1" [suppressed]
fillet "Abrundung2" [suppressed]
fillet "Abrundung3" [suppressed]
extrude "Extrusion1" [suppressed]
sketch "Skizze2" plane through (0, 0, 35) normal (0, 0, 1) x (-1, 0, 0)
  line L0 (0, -115) -> (0, 0)
  line L1 (0, 0) -> (-85, 0)
  line L2 (-85, 0) -> (-85, -115)
  line L3 (-85, -115) -> (0, -115)
  line L4 (0, 0) -> (-7, 0)
  line L5 (-7, 0) -> (-7, -7)
  line L6 (-7, -7) -> (0, -7)
  line L7 (0, -7) -> (0, 0)
  line L8 (-85, 0) -> (-78, 0)
  line L9 (-78, 0) -> (-78, -7)
  line L10 (-78, -7) -> (-85, -7)
  line L11 (-85, -7) -> (-85, 0)
  line L12 (0, -115) -> (-7, -115)
  line L13 (-7, -115) -> (-7, -108)
  line L14 (-7, -108) -> (0, -108)
  line L15 (0, -108) -> (0, -115)
  line L16 (-85, -115) -> (-78, -115)
  line L17 (-78, -115) -> (-78, -108)
  line L18 (-78, -108) -> (-85, -108)
  line L19 (-85, -108) -> (-85, -115)
  circle A0 centre (-3.5, -3.5) radius 2.65
  circle A1 centre (-81.5, -3.5) radius 2.65
  circle A2 centre (-81.5, -111.5) radius 2.65
  circle A3 centre (-3.5, -111.5) radius 2.65
  line L20 (-7, -113.25) -> (-78, -113.25)
  line L21 (-78, -113.25) -> (-78, -1.75)
  line L22 (-78, -1.75) -> (-7, -1.75)
  line L23 (-7, -1.75) -> (-7, -113.25)
  line L24 (-1.75, -108) -> (-7, -108)
  line L25 (-7, -108) -> (-7, -7)
  line L26 (-7, -7) -> (-1.75, -7)
  line L27 (-1.75, -7) -> (-1.75, -108)
  line L28 (-78, -7) -> (-83.25, -7)
  line L29 (-83.25, -7) -> (-83.25, -108)
  line L30 (-83.25, -108) -> (-78, -108)
  line L31 (-78, -108) -> (-78, -7)
  dimension "d5" = 7
  dimension "d6" = 7
  dimension "d7" = 7
  dimension "d8" = 7
  dimension "d9" = 7
  dimension "d10" = 7
  dimension "d11" = 7
  dimension "d12" = 7
  dimension "d13" = 5.3
  dimension "d14" = 5.3
  dimension "d15" = 5.3
  dimension "d16" = 5.3
  dimension "d17" = 3.5
  dimension "d18" = 3.5
  dimension "d19" = 3.5
  dimension "d20" = 3.5
  dimension "d21" = 3.5
  dimension "d22" = 3.5
  dimension "d23" = 3.5
  dimension "d24" = 3.5
  dimension "d25" = 1.75
  dimension "d26" = 1.75
  dimension "d29" = 7
  dimension "d30" = 1.75
  dimension "d31" = 7
  dimension "d32" = 7
  dimension "d33" = 7
  dimension "d34" = 1.75
  constraint horizontal L4
  constraint vertical L5
  constraint horizontal L6
  constraint vertical L7
  constraint coincident L0.end L1.start
  constraint horizontal L8
  constraint vertical L9
  constraint horizontal L10
  constraint vertical L11
  constraint coincident L1.end L2.start
  constraint horizontal L12
  constraint vertical L13
  constraint horizontal L14
  constraint vertical L15
  constraint coincident L0.start L3.end
  constraint horizontal L16
  constraint vertical L17
  constraint horizontal L18
  constraint vertical L19
  constraint coincident L2.end L3.start
  constraint horizontal L20
  constraint vertical L21
  constraint horizontal L22
  constraint vertical L23
  constraint horizontal L24
  constraint vertical L25
  constraint horizontal L26
  constraint vertical L27
  constraint coincident L23 L5.end
  constraint horizontal L28
  constraint vertical L29
  constraint horizontal L30
  constraint vertical L31
  constraint coincident L18 L29.end
  measures "d5" distance of L0.end L4.end
  measures "d6" distance of L0.end L6.end
  measures "d7" distance of L1.end L8.end
  measures "d8" distance of L1.end L10.end
  measures "d9" distance of L0.start L12.end
  measures "d10" distance of L0.start L14.end
  measures "d11" distance of L2.end L16.end
  measures "d12" distance of L2.end L18.end
  measures "d13" diameter of A0
  measures "d14" diameter of A1
  measures "d15" diameter of A2
  measures "d16" diameter of A3
  measures "d17" distance of L15 A3.centre
  measures "d18" distance of L12 A3.centre
  measures "d19" distance of L16 A2.centre
  measures "d20" distance of L19 A2.centre
  measures "d21" distance of L10 A1.centre
  measures "d22" distance of L9 A1.centre
  measures "d23" distance of L5 A0.centre
  measures "d24" distance of L6 A0.centre
  measures "d25" distance of L3 L20
  measures "d26" distance of L1 L22
  measures "d29" distance of L1 L26
  measures "d30" distance of L0 L27
  measures "d31" distance of L3 L24
  measures "d32" distance of L7 L23
  measures "d33" distance of L2 L21
  measures "d34" distance of L2 L29
extrude "Extrusion2" [suppressed]
extrude "Extrusion3" [suppressed]
extrude "Extrusion4" [suppressed]
extrude "Extrusion6" [suppressed]
equation "d35 = -30 mm + 1.75 mm"
equation "d43 = -35 mm + 1.75 mm"
equation "d69 = -30 mm + 1.75 mm"
equation "d135 = -30 mm + 1.75 mm"
